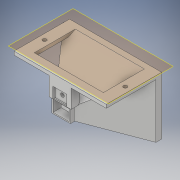
# Autodesk Inventor part: ventilador controladora
Saved by Autodesk Inventor 2019 (Build 230136000, 136)
## iProperties
Created: 2018-08-15
Part Number: ventilador controladora
Material: Genérico
Document SubType Name: Modeling
Designer: Albert Garangou Culebras
Density: 1 g/cm^3
Appearance: Valor por defecto
Author: Albert Garangou Culebras
Autodesk Inventor part; units mm, degrees
ref_plane "YZ Plane" through (0, 0, 0) normal (1, 0, 0) x (0, 1, 0)
ref_plane "XZ Plane" through (0, 0, 0) normal (0, 1, 0) x (-1, 0, 0)
ref_plane "XY Plane" through (0, 0, 0) normal (0, 0, 1) x (1, 0, 0)
sketch "Boceto1" plane through (0, 0, 0) normal (0, 0, 1) x (1, 0, 0)
  line L0 (0, 0) -> (16, 0)
  line L1 (16, 0) -> (16, -12)
  line L2 (16, -12) -> (0, -12)
  line L3 (0, -12) -> (0, 0)
  line L4 (1, -1) -> (15, -1)
  line L5 (15, -1) -> (15, -11)
  line L6 (15, -11) -> (1, -11)
  line L7 (1, -11) -> (1, -1)
  dimension "d0" = 16
  dimension "d1" = 12
  constraints: 16 end point, 4 parallel, 2 horizontal, 2 perpendicular
  measures "d0" distance of L1.end L2.end
  measures "d1" distance of L0.end L1.end
ref_plane "Plano de trabajo3" through (0, 0, -40) normal (0, 0, -1) x (-1, 0, 0)
sketch "Boceto4" plane through (0, 0, -40) normal (0, 0, -1) x (-1, 0, 0)
  line L0 (0, -12) -> (0, 0) projected
  line L1 (0, -6) -> (-16, -6)
  line L2 (-8, -31) -> (-48, -31)
  line L3 (-8, -31) -> (32, -31)
  line L4 (32, -31) -> (32, 19)
  line L5 (32, 19) -> (-48, 19)
  line L6 (-48, 19) -> (-48, -31)
  dimension "d8" = 40
  dimension "d9" = 40
  dimension "d10" = 80
  constraints: 12 end point, 2 horizontal, 1 midpoint, 1 perpendicular, 1 vertical
  measures "d8" distance of L2.start L2.end
  measures "d9" distance of L2.start L3.end
  measures "d10" distance of L4.end L5.end
extrude "Extrusión2" add sketch "Boceto1" against normal blind 40
loft "Solevación1" add profiles "Boceto4" section 1 edges at (1, -6, 0) (8, -1, 0) (15, -6, 0) (8, -11, 0)
sketch "Boceto5" plane through (0, 0, -40) normal (0, 0, -1) x (-1, 0, 0)
  line L0 (30, -29) -> (-46, -29)
  line L1 (-46, -29) -> (-46, 17)
  line L2 (-46, 17) -> (30, 17)
  line L3 (30, 17) -> (30, -29)
  point P0 (0, 0)
  constraints: 8 end point, 2 parallel, 1 horizontal, 1 perpendicular
sketch "Boceto6" plane through (0, 0, 0) normal (0, 0, 1) x (1, 0, 0)
  line L0 (1, -11) -> (15, -11)
  line L1 (15, -11) -> (15, -1)
  line L2 (15, -1) -> (1, -1)
  line L3 (1, -1) -> (1, -11)
  point P0 (0, 0)
  constraints: 8 end point, 2 parallel, 1 horizontal, 1 perpendicular
loft "Solevación2" cut profiles "Boceto6", "Boceto5"
sketch "Boceto7" plane through (0, 0, 0) normal (0, 0, 1) x (1, 0, 0)
  line L0 (0, 0) -> (16, 0) projected
  line L1 (16, -12) -> (0, -12) projected
  line L2 (0, 0) -> (16, 0)
  line L3 (16, 0) -> (16, -12)
  line L4 (16, -12) -> (0, -12)
  line L5 (0, -12) -> (0, 0)
  line L6 (1, -11) -> (1, -1) projected
  line L7 (1, -1) -> (15, -1)
  line L8 (15, -1) -> (15, -11)
  line L9 (15, -11) -> (1, -11)
  line L10 (1, -11) -> (1, -1)
  constraints: 16 end point, 4 parallel, 2 horizontal, 2 perpendicular
extrude "Extrusión3" add sketch "Boceto7" against normal blind 5
sketch "Boceto8" plane through (0, 0, 0) normal (0, 0, 1) x (1, 0, 0)
  line L0 (0, 0) -> (16, 0)
  line L1 (16, 0) -> (16, -12)
  line L2 (16, -12) -> (0, -12)
  line L3 (0, -12) -> (0, 0)
  line L4 (15, -1) -> (15, -11) projected
  line L5 (1, -1) -> (15, -1)
  line L6 (15, -1) -> (15, -11)
  line L7 (15, -11) -> (1, -11)
  line L8 (1, -11) -> (1, -1)
  constraints: 16 end point, 4 parallel, 2 horizontal, 2 perpendicular
extrude "Extrusión4" add sketch "Boceto8" along normal blind 3
ref_plane "Plano de trabajo7" through (-19.527, -29, -48.1166) normal (0.7904151, 0, -0.6125717) x (-0.6125717, 0, -0.7904151)
sketch "Boceto17" plane through (-19.527, -29, -48.1166) normal (0.7904151, 0, -0.6125717) x (-0.6125717, 0, -0.7904151)
  line L0 (-46.5554, 46) -> (0, 46) projected
  line L1 (-10.2918, 46) -> (-10.2918, 0)
  line L2 (-10.2918, 0) -> (-38.5761, 10)
  line L3 (-38.5761, 10) -> (-38, 37)
  line L4 (-38, 37) -> (-10.2918, 46)
  point P0 (-49.9938, 29)
  dimension "d37" = 30
  constraints: 8 end point, 1 point on line, 1 vertical
  measures "d37" distance of L1.end L2.end
ref_plane "Plano de trabajo8" through (35.7246, -29, -47.9634) normal (-0.7904151, 0, -0.6125717) x (-0.6125717, 0, 0.7904151)
sketch "Boceto18" plane through (35.7246, -29, -47.9634) normal (-0.7904151, 0, -0.6125717) x (-0.6125717, 0, 0.7904151)
  line L0 (0, 46) -> (46.5554, 46) projected
  line L1 (10.0792, 46) -> (10.0792, 0)
  line L2 (46.5554, 0) -> (0, 0) projected
  line L3 (10.0792, 0) -> (38.3635, 10)
  line L4 (38.3635, 10) -> (38.3635, 36)
  line L5 (38.3635, 36) -> (10.0792, 46)
  point P0 (59.7949, 29)
  dimension "d39" = 30
  constraints: 8 end point, 2 point on line, 2 vertical
  measures "d39" distance of L1.end L3.end
extrude "Extrusión9" add sketch "Boceto18" along normal blind 0.5
extrude "Extrusión10" add sketch "Boceto17" along normal blind 0.5
ref_plane "Plano de trabajo9" through (0, 19, -2) normal (0, 1, 0) x (1, 0, 0)
sketch "Boceto22" plane through (0, 19, -2) normal (0, 1, 0) x (1, 0, 0)
  line L0 (-13.199, 38) -> (-30, 38) projected
  line L1 (-30, 38) -> (13, 38) construction
  line L2 (16, -0.7879) -> (48, 38) projected
  line L3 (48, 38) -> (48, -5)
  line L4 (48, 38) -> (91, 38) construction
  line L5 (48, -5) -> (-31.7513, -5)
  line L6 (48, 38) -> (-32, 38) projected
  line L7 (-31.7513, 38) -> (-31.7513, -5)
  line L8 (-31.7513, 38) -> (11.2487, 38) construction
  line L9 (-31.7513, -5) -> (-21.7513, -5)
  line L10 (-21.7513, -5) -> (-21.7513, 38)
  line L11 (-21.7513, 38) -> (-31.7513, 38)
  line L12 (48, -5) -> (38, -5)
  line L13 (38, -5) -> (38, 38)
  line L14 (48, 38) -> (38, 38)
  point P0 (0, -2)
  dimension "d46" = 90
  dimension "d47" = 43
  dimension "d49" = 90
  dimension "d50" = 10
  dimension "d51" = 43
  dimension "d52" = 90
  dimension "d53" = 10
  dimension "d54" = 43
  constraints: 24 end point, 4 perpendicular, 4 point on line, 3 horizontal, 1 collinear
  measures "d46" angle of L3 L4
  measures "d47" distance of L2.end L3.end
  measures "d49" angle of L7 L8
  measures "d50" distance of L5.end L9.end
  measures "d51" distance of L9.end L10.end
  measures "d52" angle of L10 L9
  measures "d53" distance of L3.end L12.end
  measures "d54" distance of L12.end L13.end
extrude "Extrusión11" add sketch "Boceto22" against normal blind 3 contours L10 L5 L7 L6 L0 | L6 L2 L13 | L3 L5 L13 L2
sketch "Boceto24" plane through (38, 19, -40) normal (-1, 0, 0) x (0, 0, 1)
  line L0 (0, 0) -> (43, 0) projected
  line L1 (35.5, -2) -> (35.5, 0)
  line L2 (35.5, 0) -> (43, 0)
  line L3 (43, 0) -> (43, -2)
  line L4 (35.5, -2) -> (35.5, -3)
  line L5 (43, -3) -> (6, -3) projected
  line L6 (43, -3) -> (35.5, -3)
  line L7 (43, -3) -> (43, -2)
  line L8 (43, 0) -> (43, -3) projected
  point P0 (40, -19)
  dimension "d57" = 7.5
  constraints: 12 end point, 2 collinear, 2 point on line, 1 parallel, 1 vertical
  measures "d57" distance of L1.end L2.end
extrude "Extrusión12" add sketch "Boceto24" along normal blind 60
sketch "Boceto25" plane through (-31.7513, 19, 3) normal (0, 0, 1) x (1, 0, 0)
  line L0 (79.7513, -3) -> (0, -3) projected
  line L1 (39.8756, -3) -> (49.3756, -3)
  line L2 (39.8756, -3) -> (30.3756, -3)
  line L3 (30.3756, -3) -> (30.3756, -19)
  line L4 (30.3756, -19) -> (49.3756, -19)
  line L5 (49.3756, -19) -> (49.3756, -3)
  point P0 (31.7513, -19)
  dimension "d60" = 9.5
  dimension "d61" = 9.5
  dimension "d63" = 16
  dimension "d64" = 19
  constraints: 10 end point, 2 perpendicular, 2 point on line, 1 midpoint
  measures "d60" distance of L1.start L1.end
  measures "d61" distance of L1.start L2.end
  measures "d63" distance of L2.end L3.end
  measures "d64" distance of L3.end L4.end
extrude "Extrusión13" add sketch "Boceto25" against normal blind 7.5
sketch "Boceto27" plane through (0, 0, -40) normal (0, 0, -1) x (-1, 0, 0)
  line L0 (31.7513, 19) -> (-48, 19) projected
  line L1 (31.7513, 19) -> (-48, 19)
  line L2 (-48, 19) -> (-48, -31)
  line L3 (-48, -31) -> (31.7513, -31)
  line L4 (31.7513, -31) -> (31.7513, 19)
  line L5 (30, 16) -> (30, -29) projected
  line L6 (-46, -29) -> (-46, 16) projected
  line L7 (30, 17) -> (-46, 17)
  line L8 (-46, 17) -> (-46, -29)
  line L9 (-46, -29) -> (30, -29)
  line L10 (30, -29) -> (30, 17)
  point P0 (0, 0)
  constraints: 16 end point, 4 parallel, 2 horizontal, 2 perpendicular
extrude "Extrusión15" add sketch "Boceto27" along normal blind 5
sketch "Boceto28" plane through (0, -12, -2) normal (0, -1, 0) x (1, 0, 0)
  line L0 (16, 1) -> (0, 1)
  line L1 (0, 1) -> (0, 5)
  line L2 (0, 5) -> (16, 5)
  line L3 (16, 5) -> (16, 1)
  point P0 (0, 2)
  constraints: 8 end point, 2 parallel, 1 horizontal, 1 perpendicular
extrude "Extrusión16" add sketch "Boceto28" against normal blind 12
sketch "Boceto30" plane through (0, 0, 3) normal (0, 0, 1) x (1, 0, 0)
  line L0 (15, -11) -> (1, -11)
  line L1 (1, -11) -> (1, -1)
  line L2 (1, -1) -> (15, -1)
  line L3 (15, -1) -> (15, -11)
  point P0 (0, 0)
  constraints: 8 end point, 2 parallel, 1 horizontal, 1 perpendicular
extrude "Extrusión17" cut sketch "Boceto30" against normal blind 7.75
sketch "Boceto31" plane through (-32, -31, -40) normal (-0.7713733, 0, 0.636383) x (0.636383, 0, 0.7713733)
  line L0 (50.2239, 30.5806) -> (50.2239, 19.4194) projected
  line L1 (50.2239, 30.5806) -> (50.2239, 19.4194)
  line L2 (50.2239, 19.4194) -> (36, 14)
  line L3 (36, 14) -> (36, 36.1153)
  line L4 (50.2842, 30.6061) -> (7.7783, 47) projected
  line L5 (50.2239, 30.5806) -> (36, 36.1153)
  point P0 (51.2192, 31)
  constraints: 8 end point, 1 collinear, 1 parallel, 1 point on line
extrude "Extrusión18" add sketch "Boceto31" against normal blind 1
sketch "Boceto32" plane through (16, -11.6061, -1.2121) normal (0.7713733, 0, 0.636383) x (0.636383, 0, -0.7713733)
  line L0 (0.0603, 11.1867) -> (0.7792, 11.6061) projected
  line L1 (0.0603, -0.0001) -> (0.0603, 11.1867)
  line L2 (0.0603, 11.1867) -> (9.1306, 14.7337)
  line L3 (0, 11.2121) -> (42.5059, 27.6061) projected
  line L4 (9.1306, -0.0002) -> (9.1306, 14.7337)
  line L5 (-0.6264, 30.6061) -> (-0.6264, -19.3939) projected
  line L6 (9.1306, -0.0002) -> (9.1306, -3.5355)
  line L7 (9.1306, -3.5355) -> (0.0603, -0.0003)
  line L8 (0.0603, 0.0254) -> (0.0603, 11.1867) projected
  line L9 (0.0603, -0.0003) -> (0.0603, 11.1867)
  point P0 (-11.1171, 11.6061)
  constraints: 12 end point, 2 vertical, 1 collinear, 1 parallel, 1 point on line
extrude "Extrusión19" add sketch "Boceto32" against normal blind 1 contours L2 L4 L6 L7 L1
sketch "Boceto33" plane through (0, -12, -2) normal (0, -0.8944272, 0.4472136) x (1, 0, 0)
  line L0 (0, -0.7008) -> (0, 4.6658) projected
  line L1 (0, 0.8542) -> (-9.5417, -11.818)
  line L2 (-8.3188, -11.8619) -> (-4.3774, -6.6273) projected
  line L3 (-9.5417, -11.818) -> (25.3705, -11.818)
  line L4 (11.829, -17.3936) -> (11.829, -5.7661) projected
  line L5 (16, 0.8809) -> (19.6301, -4.0385) projected
  line L6 (25.3705, -11.818) -> (16, 0.8809)
  line L7 (16, 4.4721) -> (16, 0) projected
  line L8 (16, 0.8809) -> (16, 0)
  line L9 (16, 0) -> (0, 0)
  line L10 (0, 0) -> (0, 0.8542)
  line L11 (0, 4.4721) -> (0, 0) projected
  point P0 (0, 7.1554)
  point P1 (0, 0.0965)
  point P2 (0, 5.2759)
  constraints: 12 end point, 3 point on line, 2 collinear, 1 parallel, 1 perpendicular
extrude "Extrusión20" add sketch "Boceto33" against normal blind 1
sketch "Boceto34" plane through (0, 0, -2) normal (0, 0.8944272, 0.4472136) x (1, 0, 0)
  line L0 (30.35, 18.5661) -> (-13.525, 17.4481)
  line L1 (0, -0.8809) -> (-27.05, 35.7771) projected
  line L2 (-13.525, 17.4481) -> (0.825, -1.9989)
  line L3 (0.825, -1.9989) -> (0, -0.0364)
  line L4 (0, 0) -> (0, -0.8809) projected
  line L5 (0, 0) -> (16, 0)
  line L6 (16, 0) -> (0, 0) projected
  line L7 (16, -0.8809) -> (16, 0) projected
  line L8 (16, 0) -> (16, -0.8809)
  line L9 (16, -0.8809) -> (30.35, 18.5661)
  line L10 (16, -0.8809) -> (43.05, 35.7771) projected
  point P0 (0, -1.7889)
  point P1 (17.6244, 2.2361)
  point P2 (17.6244, 2.7951)
  constraints: 12 end point, 2 collinear, 1 midpoint, 2 other
extrude "Extrusión21" [suppressed]
sketch "Boceto35" plane through (16, -11.6061, -1.2121) normal (0.7713733, 0, 0.636383) x (0.636383, 0, -0.7713733)
  line L0 (0, 0) -> (16, -6.171)
  line L1 (9.1306, -3.5216) -> (50.2842, -19.3939) projected
  line L2 (16, -6.171) -> (16, 17.3831)
  line L3 (0, 11.2121) -> (42.5059, 27.6061) projected
  line L4 (0, 0) -> (0, 11.2121) projected
  line L5 (0, 11.2121) -> (16, 17.3831)
  line L6 (0, 11.2121) -> (0.6077, 11.6061) projected
  line L7 (0, 11.2121) -> (0, 0)
  line L8 (1.2121, 11.6061) -> (1.2121, 0.3323) projected
  point P0 (-11.1171, 11.6061)
  point P1 (1.2121, 10.8798)
  point P2 (1.2121, 0.3323)
  point P3 (0.303, 10.4264)
  point P4 (0.303, 0.7857)
  constraints: 8 end point, 2 point on line, 2 vertical, 1 other
extrude "Extrusión22" add sketch "Boceto35" against normal blind 1
sketch "Boceto37" plane through (0, 0, 3) normal (0, 0, 1) x (1, 0, 0)
  line L0 (0, -12) -> (16, -12) projected
  line L1 (0, -12) -> (16, -12)
  line L2 (16, -12) -> (16, 0)
  line L3 (16, 0) -> (0, 0)
  line L4 (0, 0) -> (0, -12)
  line L5 (1, -1) -> (15, -1) projected
  line L6 (15, -1) -> (1, -1)
  line L7 (1, -1) -> (1, -11)
  line L8 (1, -11) -> (15, -11)
  line L9 (15, -11) -> (15, -1)
  constraints: 16 end point, 4 parallel, 2 horizontal, 2 perpendicular
extrude "Extrusión23" cut sketch "Boceto37" against normal blind 1
sketch "Boceto38" plane through (-31.7513, 19, 3) normal (0, 0, 1) x (1, 0, 0)
  line L0 (30.3756, -17.75) -> (49.3756, -17.75) projected
  line L1 (30.3756, -19) -> (49.3756, -19) projected
  line L2 (39.8756, -19) -> (39.8756, -14)
  circle A0 centre (39.8756, -14) radius 1.6
  point P0 (31.7513, -19)
  dimension "d94" = 5
  dimension "d95" = 3.2
  constraints: 2 end point, 1 centre point, 1 coincident, 1 midpoint
  measures "d94" distance of L2.start L2.end
  measures "d95" diameter of A0
extrude "Extrusión24" cut sketch "Boceto38" against normal blind 11
sketch "Boceto39" plane through (-31.7513, 19, 3) normal (0, 0, 1) x (1, 0, 0)
  line L0 (34.4248, -19) -> (45.4248, -19)
  line L1 (45.4248, -9.5) -> (45.6748, -9.5)
  line L2 (45.6748, -9.5) -> (45.6748, -19)
  line L3 (16.8005, -9.5) -> (16.5505, -9.5)
  line L4 (45.6748, -19) -> (33.6748, -19)
  line L5 (45.4248, -9.5) -> (33.6748, -9.5)
  line L6 (33.6748, -19) -> (33.6748, -9.5)
  line L7 (30.3756, -17.75) -> (49.3756, -17.75) projected
  point P0 (30.3756, -3)
  point P1 (49.3756, -3)
  point P2 (16.5505, -19)
  dimension "d100" = 9.5
  dimension "d103" = 0.25
  dimension "d104" = 0.25
  dimension "d109" = 12
  constraints: 14 end point, 2 perpendicular, 1 horizontal
  measures "d100" distance of L0.end L1.start
  measures "d103" distance of L1.start L1.end
  measures "d104" distance of L3.start L3.end
  measures "d109" distance of L2.end L4.end
extrude "Extrusión25" cut sketch "Boceto39" against normal blind 2
sketch "Boceto40" plane through (0, 16, -2) normal (0, -1, 0) x (1, 0, 0)
  line L0 (-31.7513, -38) -> (-31.7513, 5) projected
  line L1 (-31.7513, 5) -> (-31.7513, -38)
  line L2 (-31.7513, -16.5) -> (-22, -16.5)
  circle A0 centre (-26.8756, -16.5) radius 1.6
  circle A1 centre (43, -16.5) radius 1.6
  point P0 (0, 2)
  dimension "d105" = 3.2
  dimension "d106" = 3.2
  constraints: 4 end point, 2 centre point, 2 midpoint, 1 collinear, 1 horizontal
  measures "d105" diameter of A0
  measures "d106" diameter of A1
extrude "Extrusión26" cut sketch "Boceto40" against normal blind 38.5
sketch "Boceto41" plane through (0, 16, -2) normal (0, -1, 0) x (1, 0, 0)
  line L0 (38, -35.7778) -> (38, -38) projected
  line L1 (38, -35.7778) -> (38, -38)
  line L2 (38, -38) -> (46, -38) projected
  line L3 (38, -38) -> (46, -38)
  line L4 (46, -38) -> (44.2885, -35.7778)
  line L5 (44.2885, -35.7778) -> (38, -35.7778)
  line L6 (-21.7513, -2.5) -> (-21.7513, -38) projected
  line L7 (-21.7513, -35.7778) -> (-21.7513, -38)
  line L8 (-30, -38) -> (-21.7513, -38) projected
  line L9 (-21.7513, -38) -> (-30, -38)
  line L10 (-30, -38) -> (-28.2778, -35.7778) projected
  line L11 (-30, -38) -> (-28.2778, -35.7778)
  line L12 (-28.2778, -35.7778) -> (-21.7513, -35.7778) projected
  line L13 (-28.2778, -35.7778) -> (-21.7513, -35.7778)
  point P0 (0, 2)
  constraints: 16 end point, 4 collinear, 2 parallel, 1 perpendicular, 1 point on line
extrude "Extrusión27" cut sketch "Boceto41" against normal blind 1
sketch "Boceto42" plane through (38, 16, -37.7778) normal (1, 0, 0) x (0, 0, -1)
  line L0 (2.2222, 1) -> (0, 1) projected
  line L1 (0, 0) -> (0, 1) projected
  line L2 (2.2222, 1) -> (0, 0)
  line L3 (0, 0) -> (0, 1)
  line L4 (0, 1) -> (2.2222, 1)
  point P0 (-37.7778, -16)
  constraints: 6 end point, 1 collinear, 1 perpendicular
sketch "Boceto43" plane through (-21.7513, 16, -37.7778) normal (-1, 0, 0) x (0, 0, 1)
  line L0 (0, 0) -> (-2.2222, 1) projected
  line L1 (-2.2222, 1) -> (0, 0)
  line L2 (0, 0) -> (0, 1) projected
  line L3 (0, 0) -> (0, 1)
  line L4 (0, 1) -> (-2.2222, 1)
  point P0 (37.7778, -16)
  constraints: 6 end point, 2 collinear, 1 perpendicular
extrude "Extrusión29" add sketch "Boceto43" along normal blind 8.75
extrude "Extrusión30" add sketch "Boceto42" along normal blind 8.25
